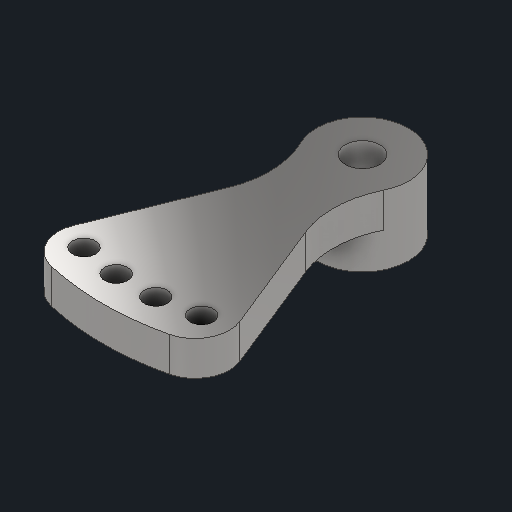
# Autodesk Inventor part: 023
Saved by Autodesk Inventor 2022 (Build 260153000, 153)
## iProperties
Created: 2021-11-21
Part Number: 023
Material: Stainless Steel, Austenitic
Document SubType Name: Modeling
Designer: vinicius.miguel
Density: 8 g/cm^3
Appearance: Semi-Polished
Author: vinicius.miguel
Autodesk Inventor part; units mm, degrees
ref_plane "YZ Plane" through (0, 0, 0) normal (1, 0, 0) x (0, 1, 0)
ref_plane "XZ Plane" through (0, 0, 0) normal (0, 1, 0) x (-1, 0, 0)
sketch "Sketch11" plane through (0, 0, 0) normal (0, 0, 1) x (1, 0, 0)
  line L0 (0, 0) -> (0, 6)
  line L1 (-4, 0) -> (-4, 3)
  line L2 (-4, 3) -> (-22.5, 3)
  line L3 (-22.5, 3) -> (-22.5, 6)
  line L4 (-22.5, 6) -> (-1.5, 6)
  line L5 (-1.5, 6) -> (-1.5, 0)
  line L6 (-1.5, 0) -> (-4, 0)
  dimension "d59" = 3
  dimension "d60" = 6
  dimension "d61" = 3
  dimension "d62" = 45
  dimension "d63" = 2.5
  constraints: 14 end point, 4 perpendicular, 2 horizontal alignment, 2 vertical, 1 parallel
  measures "d59" diameter of L5 L0
  measures "d60" distance of L4.end L5.end
  measures "d61" distance of L2.end L3.end
  measures "d62" diameter of L3 L0
  measures "d63" distance of L5.end L1.start
revolve "Revolution3" add sketch "Sketch11" angle 360 about axis through (0, 0, 0) along (0, 1, 0)
sketch "Sketch12" plane through (0, 6, 0) normal (0, 1, 0) x (1, 0, 0)
  circle A0 centre (1.7213, -19.6748) radius 1
  circle A1 centre (-1.7213, -19.6748) radius 1
  circle A2 centre (-5.1117, -19.077) radius 1
  circle A3 centre (5.1117, -19.077) radius 1
  circle A4 centre (0, 0) radius 19.75 construction
  line L0 (0, 0) -> (0, -19.75) construction
  line L1 (0, 0) -> (-1.7213, -19.6748) construction
  line L2 (0, 0) -> (-5.1117, -19.077) construction
  line L3 (0, 0) -> (1.7213, -19.6748) construction
  line L4 (0, 0) -> (5.1117, -19.077) construction
  line L5 (-5.1117, -19.077) -> (-1.7213, -19.6748) construction
  line L6 (-1.7213, -19.6748) -> (1.7213, -19.6748) construction
  dimension "d65" = 2
  dimension "d66" = 2
  dimension "d67" = 2
  dimension "d68" = 2
  dimension "d71" = 5
  dimension "d72" = 10
  dimension "d73" = 10
  dimension "d81" = 39.5
  dimension "d90" = 10.2233
  constraints: 14 end point, 5 centre point, 5 point on circle, 1 coincident, 1 perpendicular, 1 vertical
  measures "d65" diameter of A0
  measures "d66" diameter of A1
  measures "d67" diameter of A2
  measures "d68" diameter of A3
  measures "d71" angle of L0 L1
  measures "d72" angle of L2 L1
  measures "d73" angle of L4 L3
  measures "d81" diameter of A4
  measures "d90" distance of L4.end L2.end
extrude "Extrusion7" cut sketch "Sketch12" against normal through all
sketch "Sketch14" plane through (0, 6, 0) normal (0, 1, 0) x (1, 0, 0)
  circle A0 centre (0, 0) radius 22.5 projected
  line L0 (0, 0) -> (0, -22.5)
  line L1 (0, 0) -> (-8.4286, -20.8616)
  line L2 (0, 0) -> (8.4286, -20.8616)
  circle A1 centre (0, 0) radius 4 projected
  point P0 (1.4984, -3.7087)
  point P1 (-1.4984, -3.7087)
  dimension "d76" = 22
  dimension "d77" = 22
  constraints: 6 end point, 3 point on circle, 1 vertical
  measures "d76" angle of L0 L1
  measures "d77" angle of L2 L0
extrude "Extrusion8" cut sketch "Sketch14" against normal through all contours A0 L2 A1 L1
fillet "Fillet3" radius 3 2 edges at (8.4286, 4.5, 20.8616) (-8.4286, 4.5, 20.8616)
fillet "Fillet4" radius 8 2 edges at (1.4984, 4.5, 3.7087) (-1.4984, 4.5, 3.7087)
ref_plane "Work Plane2" through (0, 1.5, -4) normal (0, 0, 1) x (1, 0, 0)
sketch "Sketch15" plane through (0, 1.5, -4) normal (0, 0, 1) x (1, 0, 0)
  line L0 (4, 4.5) -> (-4, 4.5) projected
  line L1 (4, -1.5) -> (4, 4.5) projected
  point P0 (0, -1.5)
  point P1 (0, 1.5)
  point P2 (3.5894, 4.5)
  point P3 (-3.5894, 4.5)
  point P4 (0, 4.5)
  point P5 (4, 1.5)
  constraints: 2 midpoint, 1 horizontal alignment, 1 vertical alignment
hole "Hole3" at (0, 3, -4) direction (0, 0, 1) diameter 1.567 depth 4.5 tip angle 118 thread size "M2x0.4" class "6H" standard "ISO Metric profile"
equation "\"d71\" = 0.5 * d72"
equation "\"d73\" = d72"
equation "\"d77\" = d76"
body "Solid2"
